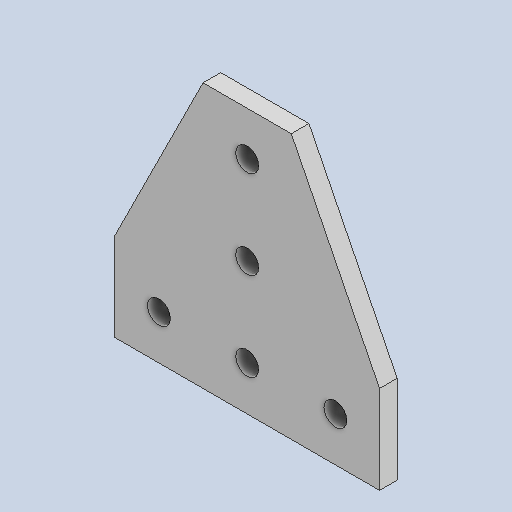
# Autodesk Inventor part: 2020 T Plate Bracket Connectors
Saved by Autodesk Inventor 2026 (Build 300175050, 175E)
## iProperties
Created: 2025-06-05
Part Number: 2020 T Plate Bracket Connectors
Material: Generic
Document SubType Name: Modeling
Designer: aadit
Density: 1 g/cm^3
Appearance: Default
Mass: 10.7753 g
Surface Area: 65.5212 cm^2
Volume: 10.7753 cm^3
Author: aadit
Autodesk Inventor part; units mm, degrees
ref_plane "YZ Plane" through (0, 0, 0) normal (1, 0, 0) x (0, 1, 0)
ref_plane "XZ Plane" through (0, 0, 0) normal (0, 1, 0) x (-1, 0, 0)
ref_plane "XY Plane" through (0, 0, 0) normal (0, 0, 1) x (1, 0, 0)
sketch "Sketch1" plane through (0, 0, 0) normal (0, 0, 1) x (1, 0, 0)
  line L0 (10, -30) -> (-10, -30)
  line L1 (-10, 30) -> (10, 30)
  line L2 (0, -30) -> (-30, -30)
  line L3 (0, -30) -> (30, -30)
  line L4 (30, -30) -> (30, -10)
  line L5 (-30, -30) -> (-30, -10)
  line L6 (-10, 30) -> (-30, -10)
  line L7 (10, 30) -> (30, -10)
  circle A0 centre (0, 0) radius 2.6
  line L8 (0, 0) -> (0, 20)
  line L9 (0, 0) -> (20, 0) construction
  circle A1 centre (0, 20) radius 2.6
  line L10 (0, 0) -> (0, -20)
  circle A2 centre (0, -20) radius 2.6
  line L11 (0, -20) -> (-20, -20)
  line L12 (0, -20) -> (20, -20) construction
  circle A3 centre (-20, -20) radius 2.6
  circle A4 centre (20, -20) radius 2.6
  dimension "d7" = 60
  dimension "d8" = 5.2
  dimension "d9" = 20
  dimension "d10" = 90
  dimension "d11" = 5.2
  dimension "d12" = 20
  dimension "d13" = 5.2
  dimension "d14" = 20
  dimension "d15" = 180
  dimension "d16" = 5.2
  dimension "d17" = 5.2
  constraints: 26 end point, 5 centre point, 5 coincident, 5 horizontal, 4 vertical, 2 equal length, 1 midpoint, 1 parallel, 1 point on line
  measures "d7" distance from line of L1 L3.end
  measures "d8" diameter of A0
  measures "d9" distance of L8.start L8.end
  measures "d10" angle of L9 L8
  measures "d11" diameter of A1
  measures "d12" distance of L8.start L10.end
  measures "d13" diameter of A2
  measures "d14" distance of L11.start L11.end
  measures "d15" angle of L11 L12
  measures "d16" diameter of A3
  measures "d17" diameter of A4
extrude "Extrusion1" add sketch "Sketch1" along normal blind 4
body "Solid1"
